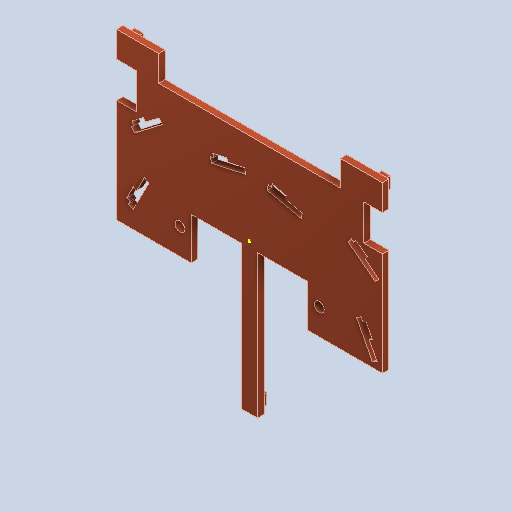
# Autodesk Inventor part: PCB
Saved by Autodesk Inventor 2022 (Build 260153000, 153)
## iProperties
Created: 2022-12-26
Part Number: PCB
Material: Copper
Document SubType Name: Modeling
Designer: Kamil
Density: 8.94 g/cm^3
Appearance: Copper - Satin
Author: Kamil
Autodesk Inventor part; units mm, degrees
(part 1 of 2)
ref_plane "YZ Plane" through (0, 0, 0) normal (1, 0, 0) x (0, 1, 0)
ref_plane "XZ Plane" through (0, 0, 0) normal (0, 1, 0) x (-1, 0, 0)
ref_plane "XY Plane" through (0, 0, 0) normal (0, 0, 1) x (1, 0, 0)
sketch "Sketch1" plane through (0, 0, 0) normal (0, 0, 1) x (1, 0, 0)
  circle A0 centre (-7.5, -8.85) radius 1.5 projected
  circle A1 centre (7.5, -8.85) radius 1.5 projected
  line L0 (50, 38.7074) -> (-50, 38.7074) projected
  line L1 (-50, 38.7074) -> (-50, -17.75) projected
  line L2 (-50, -17.75) -> (-15, -17.75) projected
  line L3 (-15, -17.75) -> (-15, -35.85) projected
  line L4 (-15, -35.85) -> (15, -35.85) projected
  line L5 (15, -35.85) -> (15, -17.75) projected
  line L6 (15, -17.75) -> (50, -17.75) projected
  line L7 (50, -17.75) -> (50, 38.7074) projected
  circle A2 centre (7.5, -26.85) radius 1.75 projected
  circle A3 centre (-7.5, -26.85) radius 1.75 projected
  line L8 (50, 31.0794) -> (-50, 31.0794) projected
  line L9 (25, 26.7074) -> (-25, 26.7074) projected
  line L10 (25, 31.0794) -> (25, 26.7074) projected
  line L11 (-25, 38.7074) -> (-25, 26.7074) projected
  line L12 (25, 26.7074) -> (25, 38.7074) projected
  line L13 (-15, -4.85) -> (-15, -48.05) projected
  line L14 (15, -4.85) -> (-15, -4.85) projected
  line L15 (15, -48.05) -> (15, -4.85) projected
  line L16 (44, 38.7074) -> (44, -17.75) projected
  line L17 (0, 26.7074) -> (0, -4.85)
  line L18 (-44, 38.7074) -> (-44, -17.75)
  point P0 (0, 0)
  constraints: 4 end point, 2 midpoint, 2 symmetric about line
extrude "Extrusion1" add sketch "Sketch1" along normal blind 2.4 contours L16 L8 L12 L0 | L16 L6 L15 L14 L17 L9 L10 L8 | L11 L8 L18 L0 | L11 L9 L17 L14 L13 L2 L18 L8
sketch "Sketch2" plane through (0, 0, 0) normal (0, 0, -1) x (-1, 0, 0)
  line L0 (-15, -4.85) -> (-15, -17.75) projected
  line L1 (-15, -17.75) -> (-44, -17.75) projected
  line L2 (-44, -17.75) -> (-44, 38.7074) projected
  line L3 (-44, 38.7074) -> (-25, 38.7074) projected
  line L4 (-25, 38.7074) -> (-25, 26.7074) projected
  line L5 (-25, 26.7074) -> (25, 26.7074) projected
  line L6 (25, 26.7074) -> (25, 38.7074) projected
  line L7 (25, 38.7074) -> (44, 38.7074) projected
  line L8 (44, 38.7074) -> (44, -17.75) projected
  line L9 (44, -17.75) -> (15, -17.75) projected
  line L10 (15, -17.75) -> (15, -4.85) projected
  line L11 (15, -4.85) -> (-15, -4.85) projected
  point P0 (0, 0)
extrude "Extrusion2" cut sketch "Sketch2" against normal blind 0.4
sketch "Sketch3" plane through (-44, -17.75, 2.4) normal (-1, 0, 0) x (0, 0, 1)
  line L0 (-2.4, 56.4574) -> (-5.4, 59.4574) projected
  line L1 (-5.4, 59.4574) -> (-5.4, 0) projected
  line L2 (-2.4, 0) -> (-5.4, 0) projected
  line L3 (-2.4, 56.4574) -> (-2.4, 0) projected
  line L4 (5.2279, 48.8294) -> (-7.5, 61.5574) projected
  line L5 (-2, 56.4574) -> (-2, 0) projected
  line L6 (-2, 0) -> (0, 0) projected
  line L7 (0, 56.4574) -> (0, 0) projected
  line L8 (-2, 56.4574) -> (0, 56.4574) projected
  line L9 (5.2279, 48.8294) -> (-2.4, 56.4574) projected
  line L10 (-2.4, 56.4574) -> (-2.4, 44.4574) projected
  line L11 (-2.4, 44.4574) -> (5.2279, 44.4574) projected
  line L12 (5.2279, 44.4574) -> (5.2279, 48.8294) projected
  line L13 (-2, 56.4574) -> (-2, 44.4574) projected
  line L14 (-2, 48.8294) -> (0, 48.8294)
  line L15 (0, 0) -> (0, 56.4574) projected
  line L16 (0, 50.4574) -> (-2, 50.4574)
  point P0 (-2.4, 17.75)
  constraints: 4 end point, 3 point on line, 1 midpoint, 1 perpendicular
extrude "Extrusion3" cut sketch "Sketch3" against normal through all contours L5 L8 L7 L4 | L4 L7 L16 L5
sketch "Sketch4" plane through (0, 0, 0.4) normal (0, 0, -1) x (-1, 0, 0)
  line L0 (-3.5, -4.85) -> (-3.5, -48.05) projected
  line L1 (3.5, -48.05) -> (3.5, -4.85) projected
  line L2 (5.6525, -48.05) -> (-5.6525, -48.05) projected
  line L3 (-44, 32.7074) -> (-25, 32.7074) projected
  line L4 (-25, 32.7074) -> (-25, 26.7074) projected
  line L5 (-25, 26.7074) -> (25, 26.7074) projected
  line L6 (25, 26.7074) -> (25, 32.7074) projected
  line L7 (25, 32.7074) -> (44, 32.7074) projected
  line L8 (44, 32.7074) -> (44, -17.75) projected
  line L9 (44, -17.75) -> (15, -17.75) projected
  line L10 (15, -17.75) -> (15, -4.85) projected
  line L11 (15, -4.85) -> (-15, -4.85) projected
  line L12 (-15, -4.85) -> (-15, -17.75) projected
  line L13 (-15, -17.75) -> (-44, -17.75) projected
  line L14 (-44, -17.75) -> (-44, 32.7074) projected
  point P0 (0, 0)
extrude "Extrusion4" add sketch "Sketch4" against normal blind 2 contours L11 L1 L2 L0
sketch "Sketch5" plane through (0, 0, 2.4) normal (0, 0, 1) x (1, 0, 0)
  line L0 (44, 32.7074) -> (25, 32.7074) projected
  line L1 (25, 32.7074) -> (25, 26.7074) projected
  line L2 (25, 26.7074) -> (-25, 26.7074) projected
  line L3 (-25, 26.7074) -> (-25, 32.7074) projected
  line L4 (-25, 32.7074) -> (-44, 32.7074) projected
  line L5 (-44, 32.7074) -> (-44, -17.75) projected
  line L6 (-44, -17.75) -> (-15, -17.75) projected
  line L7 (-15, -17.75) -> (-15, -4.85) projected
  line L8 (-15, -4.85) -> (-3.5, -4.85) projected
  line L9 (-3.5, -4.85) -> (-3.5, -48.05) projected
  line L10 (-3.5, -48.05) -> (3.5, -48.05) projected
  line L11 (3.5, -48.05) -> (3.5, -4.85) projected
  line L12 (3.5, -4.85) -> (15, -4.85) projected
  line L13 (15, -4.85) -> (15, -17.75) projected
  line L14 (15, -17.75) -> (44, -17.75) projected
  line L15 (44, -17.75) -> (44, 32.7074) projected
  line L16 (-25, 31.0794) -> (25, 31.0794) projected
  point P0 (0, 0)
extrude "Extrusion5" add sketch "Sketch5" against normal blind 2 contours L1 L2 L3 L16
sketch "Sketch6" plane through (0, 0, 2.4) normal (0, 0, 1) x (1, 0, 0)
  line L0 (44, 32.7074) -> (25, 32.7074) projected
  line L1 (25, 32.7074) -> (25, 31.0794) projected
  line L2 (25, 31.0794) -> (-25, 31.0794) projected
  line L3 (-25, 31.0794) -> (-25, 32.7074) projected
  line L4 (-25, 32.7074) -> (-44, 32.7074) projected
  line L5 (-44, 32.7074) -> (-44, -17.75) projected
  line L6 (-44, -17.75) -> (-15, -17.75) projected
  line L7 (-15, -17.75) -> (-15, -4.85) projected
  line L8 (-15, -4.85) -> (-3.5, -4.85) projected
  line L9 (-3.5, -4.85) -> (-3.5, -48.05) projected
  line L10 (-3.5, -48.05) -> (3.5, -48.05) projected
  line L11 (3.5, -48.05) -> (3.5, -4.85) projected
  line L12 (3.5, -4.85) -> (15, -4.85) projected
  line L13 (15, -4.85) -> (15, -17.75) projected
  line L14 (15, -17.75) -> (44, -17.75) projected
  line L15 (44, -17.75) -> (44, 32.7074) projected
  line L16 (25, 32.7074) -> (25, 31.0794) projected
  line L17 (25, 32.7074) -> (44, 32.7074)
  line L18 (44, 32.7074) -> (44, 36.1074)
  line L19 (44, 36.1074) -> (25, 36.1074)
  line L20 (25, 36.1074) -> (25, 32.7074)
  line L21 (-44, 32.7074) -> (-25, 32.7074) projected
  line L22 (-44, 32.7074) -> (-25, 32.7074)
  line L23 (-25, 32.7074) -> (-25, 36.1074)
  line L24 (-25, 36.1074) -> (-44, 36.1074)
  line L25 (-44, 36.1074) -> (-44, 32.7074)
  point P0 (0, 0)
  dimension "d10" = 3.4
  constraints: 16 end point, 4 parallel, 2 horizontal, 2 perpendicular, 1 point on line
  measures "d10" distance of L18.end L17.end
extrude "Extrusion6" add sketch "Sketch6" against normal blind 2 contours L0 L20 L19 L18 | L4 L25 L24 L23
sketch "Sketch9" plane through (0, 0, 2.4) normal (0, 0, 1) x (1, 0, 0)
  line L0 (44, -17.75) -> (44, 36.1074) projected
  line L1 (44, 33.1074) -> (44, 36.1074)
  line L2 (15, -17.75) -> (44, -17.75) projected
  line L3 (44, 36.1074) -> (41, 36.1074)
  line L4 (41, 36.1074) -> (41, -17.75)
  line L5 (41, -17.75) -> (44, -17.75)
  line L6 (44, -17.75) -> (44, 36.1074)
  line L7 (-44, 36.1074) -> (-44, -17.75) projected
  line L8 (44, -17.75) -> (-44, -17.75)
  line L9 (-44, -17.75) -> (-44, -13.0168)
  line L10 (-44, -13.0168) -> (44, -13.0168)
  line L11 (44, -13.0168) -> (44, -17.75)
  line L12 (15, -4.85) -> (15, -17.75) projected
  line L13 (15, -17.75) -> (18, -17.75)
  line L14 (18, -17.75) -> (18, -4.85)
  line L15 (18, -4.85) -> (15, -4.85)
  line L16 (15, -4.85) -> (15, -17.75)
  line L17 (-15, -17.75) -> (-15, -4.85) projected
  line L18 (-15, -17.75) -> (-18, -17.75)
  line L19 (-18, -17.75) -> (-18, -4.85)
  line L20 (-18, -4.85) -> (-15, -4.85)
  line L21 (-15, -4.85) -> (-15, -17.75)
  line L22 (-25, 36.1074) -> (-44, 36.1074) projected
  line L23 (-44, -17.75) -> (-41, -17.75)
  line L24 (-41, -17.75) -> (-41, 36.1074)
  line L25 (-41, 36.1074) -> (-44, 36.1074)
  line L26 (-44, 36.1074) -> (-44, -17.75)
  line L27 (25, 36.1074) -> (25, 31.0794) projected
  line L28 (25, 36.1074) -> (28, 36.1074)
  line L29 (28, 36.1074) -> (28, 31.0794)
  line L30 (28, 31.0794) -> (25, 31.0794)
  line L31 (25, 31.0794) -> (25, 36.1074)
  line L32 (-25, 36.1074) -> (-28, 36.1074)
  line L33 (-28, 36.1074) -> (-28, 31.0794)
  line L34 (-28, 31.0794) -> (-25, 31.0794)
  line L35 (-25, 31.0794) -> (-25, 36.1074)
  line L36 (-18, -4.85) -> (-3.5, -4.85)
  line L37 (-3.5, -4.85) -> (-3.5, -1.85)
  line L38 (-3.5, -1.85) -> (-18, -1.85)
  line L39 (-18, -1.85) -> (-18, -4.85)
  line L40 (3.5, -48.05) -> (3.5, -4.85) projected
  line L41 (3.5, -4.85) -> (18, -4.85)
  line L42 (18, -4.85) -> (18, -1.85)
  line L43 (18, -1.85) -> (3.5, -1.85)
  line L44 (3.5, -1.85) -> (3.5, -4.85)
  line L45 (-3.5, -48.05) -> (3.5, -48.05) projected
  line L46 (3.5, -1.85) -> (2.5, -1.85)
  line L47 (2.5, -1.85) -> (2.5, -48.05)
  line L48 (2.5, -48.05) -> (3.5, -48.05)
  line L49 (3.5, -48.05) -> (3.5, -1.85)
  line L50 (-3.5, -48.05) -> (-2.5, -48.05)
  line L51 (-2.5, -48.05) -> (-2.5, -4.85)
  line L52 (-2.5, -4.85) -> (-3.5, -4.85)
  line L53 (-3.5, -4.85) -> (-3.5, -48.05)
  line L54 (-28, 31.0794) -> (28, 31.0794)
  line L55 (28, 31.0794) -> (28, 28.0794)
  line L56 (28, 28.0794) -> (-28, 28.0794)
  line L57 (-28, 28.0794) -> (-28, 31.0794)
  point P0 (0, 0)
  point P1 (-18, -13.0168)
  point P2 (-41, -13.0168)
  point P3 (41, -13.0168)
  point P4 (18, -13.0168)
  dimension "d14" = 3
  dimension "d15" = 3
  dimension "d16" = 3
  dimension "d17" = 3
  dimension "d18" = 3
  dimension "d19" = 3
  dimension "d20" = 3
  dimension "d21" = 1
  dimension "d22" = 1
  dimension "d23" = 3
  constraints: 98 end point, 24 parallel, 12 horizontal, 12 perpendicular, 9 point on line
  measures "d14" distance of L5.end L4.end
  measures "d15" distance of L15.end L14.end
  measures "d16" distance of L19.end L20.end
  measures "d17" distance of L25.end L24.end
  measures "d18" distance of L29.end L30.end
  measures "d19" distance of L34.end L33.end
  measures "d20" distance of L37.end L36.end
  measures "d21" distance of L48.end L47.end
  measures "d22" distance of L52.end L51.end
  measures "d23" distance of L54.end L55.end
extrude "Extrusion7" cut sketch "Sketch9" against normal blind 2 contours L2 L4 L10 L0 | L22 L35 L34 L33 | L10 L4 L3 L0 | L2 L14 L10 L4 | L2 L12 L10 L14 | L10 L12 L15 L14 | L15 L41 L44 L43 L42 | L40 L45 L47 L8 | L8 L47 L10 L40 | L10 L47 L46 L44 L40 | L51 L45 L53 L8 | L8 L53 L10 L51 | L10 L53 L52 L51 | L8 L19 L10 L17 | L10 L19 L20 L17 | L36 L20 L39 L38 L37 | L8 L24 L10 L19 | L8 L7 L10 L24 | L10 L7 L22 L24 | L34 L54 L30 L55 L56 L57 | L27 L28 L29 L30
sketch "Sketch8" plane through (0, 0, 2.4) normal (0, 0, 1) x (1, 0, 0)
  line L0 (-40.8006, -12.2713) -> (-38.4785, -1.8263)
  line L1 (-40.8006, -12.2713) -> (-39.2388, -12.6185)
  line L2 (-36.9167, -2.1735) -> (-39.2388, -12.6185)
  line L3 (-38.4785, -1.8263) -> (-36.9167, -2.1735)
  line L4 (36.1788, 2.3275) -> (38.4885, -8.1203)
  line L5 (36.1788, 2.3275) -> (34.6166, 1.9821)
  line L6 (36.9263, -8.4656) -> (34.6166, 1.9821)
  line L7 (38.4885, -8.1203) -> (36.9263, -8.4656)
  line L8 (-3.9031, 21.0008) -> (-14.3503, 18.6891)
  line L9 (-3.9031, 21.0008) -> (-3.5574, 19.4386)
  line L10 (-14.0047, 17.1269) -> (-3.5574, 19.4386)
  line L11 (-14.3503, 18.6891) -> (-14.0047, 17.1269)
  line L12 (9.235, 18.6922) -> (-1.2105, 21.0122)
  line L13 (9.235, 18.6922) -> (8.888, 17.1302)
  line L14 (-1.5574, 19.4503) -> (8.888, 17.1302)
  line L15 (-1.2105, 21.0122) -> (-1.5574, 19.4503)
  line L16 (-39.7739, 3.0399) -> (-32.2458, 10.6437)
  line L17 (-39.7739, 3.0399) -> (-38.6369, 1.9142)
  line L18 (-31.1088, 9.5181) -> (-38.6369, 1.9142)
  line L19 (-32.2458, 10.6437) -> (-31.1088, 9.5181)
  line L20 (32.5559, 15.107) -> (40.1958, 7.6154)
  line L21 (32.5559, 15.107) -> (31.4357, 13.9645)
  line L22 (39.0755, 6.473) -> (31.4357, 13.9645)
  line L23 (40.1958, 7.6154) -> (39.0755, 6.473)
  line L24 (25, 36.1074) -> (25, 31.0794)
  line L25 (25, 31.0794) -> (-25, 31.0794)
  line L26 (-25, 31.0794) -> (-25, 36.1074)
  line L27 (-25, 36.1074) -> (-44, 36.1074)
  line L28 (-44, 36.1074) -> (-44, -17.75)
  line L29 (-44, -17.75) -> (-15, -17.75)
  line L30 (-15, -17.75) -> (-15, -4.85)
  line L31 (-15, -4.85) -> (-3.5, -4.85)
  line L32 (-3.5, -4.85) -> (-3.5, -48.05)
  line L33 (-3.5, -48.05) -> (3.5, -48.05)
  line L34 (3.5, -48.05) -> (3.5, -4.85)
  line L35 (3.5, -4.85) -> (15, -4.85)
  line L36 (15, -4.85) -> (15, -17.75)
  line L37 (15, -17.75) -> (44, -17.75)
  line L38 (44, -17.75) -> (44, 36.1074)
  line L39 (44, 36.1074) -> (25, 36.1074)
  point P0 (0, 0)
extrude "Extrusion8" add sketch "Sketch8" along normal blind 14 contours L0 L3 L2 L1 | L4 L7 L6 L5 | L9 L10 L11 L8 | L13 L14 L15 L12 | L16 L19 L18 L17 | L20 L23 L22 L21
sketch "Sketch10" plane through (0, 0, 2.4) normal (0, 0, 1) x (1, 0, 0)
  line L0 (-1.2105, 21.0122) -> (9.235, 18.6922) projected
  line L1 (9.235, 18.6922) -> (8.888, 17.1302) projected
  line L2 (8.888, 17.1302) -> (-1.5574, 19.4503) projected
  line L3 (-1.5574, 19.4503) -> (-1.2105, 21.0122) projected
  line L4 (-39.2388, -12.6185) -> (-40.8006, -12.2713) projected
  line L5 (-40.8006, -12.2713) -> (-38.4785, -1.8263) projected
  line L6 (-38.4785, -1.8263) -> (-36.9167, -2.1735) projected
  line L7 (-36.9167, -2.1735) -> (-39.2388, -12.6185) projected
  line L8 (34.6166, 1.9821) -> (36.1788, 2.3275) projected
  line L9 (36.1788, 2.3275) -> (38.4885, -8.1203) projected
  line L10 (38.4885, -8.1203) -> (36.9263, -8.4656) projected
  line L11 (36.9263, -8.4656) -> (34.6166, 1.9821) projected
  line L12 (-14.3503, 18.6891) -> (-3.9031, 21.0008) projected
  line L13 (-3.9031, 21.0008) -> (-3.5574, 19.4386) projected
  line L14 (-3.5574, 19.4386) -> (-14.0047, 17.1269) projected
  line L15 (-14.0047, 17.1269) -> (-14.3503, 18.6891) projected
  line L16 (-38.6369, 1.9142) -> (-39.7739, 3.0399) projected
  line L17 (-39.7739, 3.0399) -> (-32.2458, 10.6437) projected
  line L18 (-32.2458, 10.6437) -> (-31.1088, 9.5181) projected
  line L19 (-31.1088, 9.5181) -> (-38.6369, 1.9142) projected
  line L20 (31.4357, 13.9645) -> (32.5559, 15.107) projected
  line L21 (32.5559, 15.107) -> (40.1958, 7.6154) projected
  line L22 (40.1958, 7.6154) -> (39.0755, 6.473) projected
  line L23 (39.0755, 6.473) -> (31.4357, 13.9645) projected
  line L24 (28, 36.1074) -> (28, 28.0794) projected
  line L25 (28, 28.0794) -> (-28, 28.0794) projected
  line L26 (-28, 28.0794) -> (-28, 36.1074) projected
  line L27 (-28, 36.1074) -> (-41, 36.1074) projected
  line L28 (-41, 36.1074) -> (-41, -13.0168) projected
  line L29 (-41, -13.0168) -> (-18, -13.0168) projected
  line L30 (-18, -13.0168) -> (-18, -1.85) projected
  line L31 (-18, -1.85) -> (-3.5, -1.85) projected
  line L32 (-3.5, -1.85) -> (-3.5, -4.85) projected
  line L33 (-3.5, -4.85) -> (-2.5, -4.85) projected
  line L34 (-2.5, -4.85) -> (-2.5, -48.05) projected
  line L35 (-2.5, -48.05) -> (2.5, -48.05) projected
  line L36 (2.5, -48.05) -> (2.5, -1.85) projected
  line L37 (2.5, -1.85) -> (18, -1.85) projected
  line L38 (18, -1.85) -> (18, -13.0168) projected
  line L39 (18, -13.0168) -> (41, -13.0168) projected
  line L40 (41, -13.0168) -> (41, 36.1074) projected
  line L41 (41, 36.1074) -> (28, 36.1074) projected
  line L42 (-3.5, -4.85) -> (-2.5, -4.85)
  line L43 (-2.5, -4.85) -> (-2.5, -1.85)
  line L44 (-2.5, -1.85) -> (-3.5, -1.85)
  line L45 (-3.5, -1.85) -> (-3.5, -4.85)
  point P0 (0, 0)
  constraints: 8 end point, 2 parallel, 1 horizontal, 1 perpendicular
extrude "Extrusion9" cut sketch "Sketch10" against normal blind 14 contours L44 L43 L33 L32
sketch "Sketch11" plane through (0, 0, 2.4) normal (0, 0, 1) x (1, 0, 0)
  line L0 (-2.5, -1.85) -> (-2.5, -48.05) projected
  line L1 (-2.5, -48.05) -> (2.5, -48.05) projected
  line L2 (2.5, -48.05) -> (2.5, -1.85) projected
  line L3 (2.5, -1.85) -> (18, -1.85) projected
  line L4 (18, -1.85) -> (18, -13.0168) projected
  line L5 (18, -13.0168) -> (41, -13.0168) projected
  line L6 (41, -13.0168) -> (41, 36.1074) projected
  line L7 (41, 36.1074) -> (28, 36.1074) projected
  line L8 (28, 36.1074) -> (28, 28.0794) projected
  line L9 (28, 28.0794) -> (-28, 28.0794) projected
  line L10 (-28, 28.0794) -> (-28, 36.1074) projected
  line L11 (-28, 36.1074) -> (-41, 36.1074) projected
  line L12 (-41, 36.1074) -> (-41, -13.0168) projected
  line L13 (-41, -13.0168) -> (-18, -13.0168) projected
  line L14 (-18, -13.0168) -> (-18, -1.85) projected
  line L15 (-18, -1.85) -> (-2.5, -1.85) projected
  line L16 (-1.2105, 21.0122) -> (9.235, 18.6922) projected
  line L17 (9.235, 18.6922) -> (8.888, 17.1302) projected
  line L18 (8.888, 17.1302) -> (-1.5574, 19.4503) projected
  line L19 (-1.5574, 19.4503) -> (-1.2105, 21.0122) projected
  line L20 (-39.2388, -12.6185) -> (-40.8006, -12.2713) projected
  line L21 (-40.8006, -12.2713) -> (-38.4785, -1.8263) projected
  line L22 (-38.4785, -1.8263) -> (-36.9167, -2.1735) projected
  line L23 (-36.9167, -2.1735) -> (-39.2388, -12.6185) projected
  line L24 (34.6166, 1.9821) -> (36.1788, 2.3275) projected
  line L25 (36.1788, 2.3275) -> (38.4885, -8.1203) projected
  line L26 (38.4885, -8.1203) -> (36.9263, -8.4656) projected
  line L27 (36.9263, -8.4656) -> (34.6166, 1.9821) projected
  line L28 (-14.3503, 18.6891) -> (-3.9031, 21.0008) projected
  line L29 (-3.9031, 21.0008) -> (-3.5574, 19.4386) projected
  line L30 (-3.5574, 19.4386) -> (-14.0047, 17.1269) projected
  line L31 (-14.0047, 17.1269) -> (-14.3503, 18.6891) projected
  line L32 (-38.6369, 1.9142) -> (-39.7739, 3.0399) projected
  line L33 (-39.7739, 3.0399) -> (-32.2458, 10.6437) projected
  line L34 (-32.2458, 10.6437) -> (-31.1088, 9.5181) projected
  line L35 (-31.1088, 9.5181) -> (-38.6369, 1.9142) projected
  line L36 (31.4357, 13.9645) -> (32.5559, 15.107) projected
  line L37 (32.5559, 15.107) -> (40.1958, 7.6154) projected
  line L38 (40.1958, 7.6154) -> (39.0755, 6.473) projected
  line L39 (39.0755, 6.473) -> (31.4357, 13.9645) projected
  line L40 (0, -48.05) -> (0, 28.0794)
  line L41 (28, 28.0794) -> (-28, 28.0794) projected
  line L42 (41, -13.0168) -> (41, 36.1074) projected
  line L43 (41, 28.0794) -> (35.2556, 28.0794)
  line L44 (35.2556, 28.0794) -> (35.2556, 17.8601)
  line L45 (35.2556, 17.8601) -> (41, 17.8601)
  line L46 (41, 17.8601) -> (41, 28.0794)
  line L47 (-41, 28.0794) -> (-35.2556, 28.0794)
  line L48 (-35.2556, 28.0794) -> (-35.2556, 17.8601)
  line L49 (-35.2556, 17.8601) -> (-41, 17.8601)
  point P0 (0, 0)
  constraints: 16 end point, 4 symmetric about line, 2 midpoint, 2 parallel, 1 horizontal, 1 perpendicular, 1 point on line
extrude "Extrusion10" cut sketch "Sketch11" against normal blind 14 contours L12 L47 L48 L49 | L45 L44 L43 L6
sketch "Sketch12" plane through (0, 0, 2.4) normal (0, 0, 1) x (1, 0, 0)
  line L0 (31.4357, 13.9645) -> (32.5559, 15.107) projected
  line L1 (32.5559, 15.107) -> (40.1958, 7.6154) projected
  line L2 (40.1958, 7.6154) -> (39.0755, 6.473) projected
  line L3 (39.0755, 6.473) -> (31.4357, 13.9645) projected
  line L4 (-38.6369, 1.9142) -> (-39.7739, 3.0399) projected
  line L5 (-39.7739, 3.0399) -> (-32.2458, 10.6437) projected
  line L6 (-32.2458, 10.6437) -> (-31.1088, 9.5181) projected
  line L7 (-31.1088, 9.5181) -> (-38.6369, 1.9142) projected
  line L8 (-14.3503, 18.6891) -> (-3.9031, 21.0008) projected
  line L9 (-3.9031, 21.0008) -> (-3.5574, 19.4386) projected
  line L10 (-3.5574, 19.4386) -> (-14.0047, 17.1269) projected
  line L11 (-14.0047, 17.1269) -> (-14.3503, 18.6891) projected
  line L12 (34.6166, 1.9821) -> (36.1788, 2.3275) projected
  line L13 (36.1788, 2.3275) -> (38.4885, -8.1203) projected
  line L14 (38.4885, -8.1203) -> (36.9263, -8.4656) projected
  line L15 (36.9263, -8.4656) -> (34.6166, 1.9821) projected
  line L16 (-39.2388, -12.6185) -> (-40.8006, -12.2713) projected
  line L17 (-40.8006, -12.2713) -> (-38.4785, -1.8263) projected
  line L18 (-38.4785, -1.8263) -> (-36.9167, -2.1735) projected
  line L19 (-36.9167, -2.1735) -> (-39.2388, -12.6185) projected
  line L20 (-1.2105, 21.0122) -> (9.235, 18.6922) projected
  line L21 (9.235, 18.6922) -> (8.888, 17.1302) projected
  line L22 (8.888, 17.1302) -> (-1.5574, 19.4503) projected
  line L23 (-1.5574, 19.4503) -> (-1.2105, 21.0122) projected
  line L24 (-41, 28.0794) -> (-35.2556, 28.0794) projected
  line L25 (-35.2556, 28.0794) -> (-35.2556, 17.8601) projected
  line L26 (-35.2556, 17.8601) -> (-41, 17.8601) projected
  line L27 (-41, 17.8601) -> (-41, -13.0168) projected
  line L28 (-41, -13.0168) -> (-18, -13.0168) projected
  line L29 (-18, -13.0168) -> (-18, -1.85) projected
  line L30 (-18, -1.85) -> (-2.5, -1.85) projected
  line L31 (-2.5, -1.85) -> (-2.5, -48.05) projected
  line L32 (-2.5, -48.05) -> (2.5, -48.05) projected
  line L33 (2.5, -48.05) -> (2.5, -1.85) projected
  line L34 (2.5, -1.85) -> (18, -1.85) projected
  line L35 (18, -1.85) -> (18, -13.0168) projected
  line L36 (18, -13.0168) -> (41, -13.0168) projected
  line L37 (41, -13.0168) -> (41, 17.8601) projected
  line L38 (41, 17.8601) -> (35.2556, 17.8601) projected
  line L39 (35.2556, 17.8601) -> (35.2556, 28.0794) projected
  line L40 (35.2556, 28.0794) -> (41, 28.0794) projected
  line L41 (41, 28.0794) -> (41, 36.1074) projected
  line L42 (41, 36.1074) -> (28, 36.1074) projected
  line L43 (28, 36.1074) -> (28, 28.0794) projected
  line L44 (28, 28.0794) -> (-28, 28.0794) projected
  line L45 (-28, 28.0794) -> (-28, 36.1074) projected
  line L46 (-28, 36.1074) -> (-41, 36.1074) projected
  line L47 (-41, 36.1074) -> (-41, 28.0794) projected
  line L48 (-1.5574, 19.4503) -> (-1.2105, 21.0122) projected
  line L49 (-1.5574, 19.4503) -> (-1.5574, 15.4503)
  line L50 (-1.5574, 19.4503) -> (8.888, 17.1302) projected
  line L51 (9.235, 18.6922) -> (-1.2105, 21.0122) projected
  line L52 (-1.2105, 21.0122) -> (-1.5574, 19.4503) projected
  line L53 (-1.5574, 19.4503) -> (8.888, 17.1302) projected
  line L54 (8.888, 17.1302) -> (9.235, 18.6922) projected
  line L55 (9.235, 18.6922) -> (-1.2105, 21.0122) projected
  line L56 (-14.3503, 18.6891) -> (-14.0047, 17.1269) projected
  line L57 (-14.0047, 17.1269) -> (-3.5574, 19.4386) projected
  line L58 (-3.5574, 19.4386) -> (-3.9031, 21.0008) projected
  line L59 (-3.9031, 21.0008) -> (-14.3503, 18.6891) projected
  line L60 (-1.5574, 17.4503) -> (8.888, 15.1302)
  line L61 (9.235, 18.6922) -> (8.888, 17.1302) projected
  line L62 (-1.2105, 21.0122) -> (9.235, 18.6922) projected
  line L63 (9.235, 16.6922) -> (-1.2105, 19.0122)
  line L64 (-1.2105, 19.0122) -> (-1.5574, 17.4503)
  line L65 (-3.9031, 21.0008) -> (-3.5574, 19.4386) projected
  line L66 (-14.0047, 17.1269) -> (-14.3503, 18.6891) projected
  line L67 (-3.9031, 19.0008) -> (-14.3503, 16.6891)
  line L68 (-14.3503, 16.6891) -> (-14.0047, 15.1269)
  line L69 (-14.0047, 15.1269) -> (-3.5574, 17.4386)
  line L70 (-3.5574, 19.4386) -> (-14.0047, 17.1269) projected
  line L71 (-3.5574, 17.4386) -> (-3.9031, 19.0008)
  line L72 (8.888, 15.1302) -> (9.235, 16.6922)
  line L73 (12.4945, 18.6922) -> (12.4945, 16.6922)
  point P0 (0, 0)
  point P1 (-3.5574, 17.4386)
  dimension "d33" = 2
  constraints: 20 end point, 4 perpendicular, 3 parallel, 2 vertical
  measures "d33" distance of L73.start L73.end
extrude "Extrusion11" add sketch "Sketch12" along normal blind 14 contours L64 L63 L72 L60 | L71 L69 L68 L67
extrude "Extrusion12" cut sketch "Sketch12" along normal blind 14 contours L8 L9 L10 L11 | L20 L21 L22 L23
sketch "Sketch13" plane through (0, 0, 0.4) normal (0, 0, -1) x (-1, 0, 0)
  line L0 (41, 17.8601) -> (35.2556, 17.8601) projected
  line L1 (35.2556, 17.8601) -> (35.2556, 28.0794) projected
  line L2 (35.2556, 28.0794) -> (41, 28.0794) projected
  line L3 (41, 28.0794) -> (41, 36.1074) projected
  line L4 (41, 36.1074) -> (28, 36.1074) projected
  line L5 (28, 36.1074) -> (28, 28.0794) projected
  line L6 (28, 28.0794) -> (-28, 28.0794) projected
  line L7 (-28, 28.0794) -> (-28, 36.1074) projected
  line L8 (-28, 36.1074) -> (-41, 36.1074) projected
  line L9 (-41, 36.1074) -> (-41, 28.0794) projected
  line L10 (-41, 28.0794) -> (-35.2556, 28.0794) projected
  line L11 (-35.2556, 28.0794) -> (-35.2556, 17.8601) projected
  line L12 (-35.2556, 17.8601) -> (-41, 17.8601) projected
  line L13 (-41, 17.8601) -> (-41, -13.0168) projected
  line L14 (-41, -13.0168) -> (-18, -13.0168) projected
  line L15 (-18, -13.0168) -> (-18, -1.85) projected
  line L16 (-18, -1.85) -> (-2.5, -1.85) projected
  line L17 (-2.5, -1.85) -> (-2.5, -48.05) projected
  line L18 (-2.5, -48.05) -> (2.5, -48.05) projected
  line L19 (2.5, -48.05) -> (2.5, -1.85) projected
  line L20 (2.5, -1.85) -> (18, -1.85) projected
  line L21 (18, -1.85) -> (18, -13.0168) projected
  line L22 (18, -13.0168) -> (41, -13.0168) projected
  line L23 (41, -13.0168) -> (41, 17.8601) projected
  line L24 (2.5, -1.85) -> (2.5, -48.05) projected
  line L25 (-2.5, -48.05) -> (2.5, -48.05)
  line L26 (2.5, -48.05) -> (2.5, -46.05)
  line L27 (2.5, -46.05) -> (-2.5, -46.05)
  line L28 (-2.5, -46.05) -> (-2.5, -48.05)
  point P0 (0, 0)
  dimension "d38" = 2
  constraints: 8 end point, 2 parallel, 1 horizontal, 1 perpendicular, 1 point on line
  measures "d38" distance of L26.end L25.end
extrude "Extrusion13" cut sketch "Sketch13" against normal blind 14 contours L19 L18 L17 L27
sketch "Sketch14" plane through (0, 0, 2.4) normal (0, 0, 1) x (1, 0, 0)
  circle A0 centre (21.5, -6.85) radius 1.5 projected
  circle A1 centre (-21.5, -6.85) radius 1.5 projected
  circle A2 centre (7.5, -24.85) radius 1.75 projected
  circle A3 centre (-7.5, -24.85) radius 1.75 projected
  circle A4 centre (7.5, -6.85) radius 1.5 projected
  circle A5 centre (-7.5, -6.85) radius 1.5 projected
  line L0 (-50, 42.8801) -> (50, 42.8801) projected
  line L1 (50, -15.75) -> (50, 42.8801) projected
  line L2 (15, -15.75) -> (50, -15.75) projected
  line L3 (15, -33.85) -> (15, -15.75) projected
  line L4 (15, -33.85) -> (-15, -33.85) projected
  line L5 (-15, -15.75) -> (-15, -33.85) projected
  line L6 (-50, -15.75) -> (-15, -15.75) projected
  line L7 (-50, 42.8801) -> (-50, -15.75) projected
  point P0 (0, 0)
extrude "Extrusion14" cut sketch "Sketch14" against normal blind 14 contours A0 | A1
sketch "Sketch15" plane through (0, 0, 0.4) normal (0, 0, -1) x (-1, 0, 0)
  circle A0 centre (21.5, -6.85) radius 1.5 projected
  circle A1 centre (-21.5, -6.85) radius 1.5 projected
  line L0 (-2.5, -46.05) -> (2.5, -46.05) projected
  line L1 (2.5, -46.05) -> (2.5, -1.85) projected
  line L2 (2.5, -1.85) -> (18, -1.85) projected
  line L3 (18, -1.85) -> (18, -13.0168) projected
  line L4 (18, -13.0168) -> (41, -13.0168) projected
  line L5 (41, -13.0168) -> (41, 17.8601) projected
  line L6 (41, 17.8601) -> (35.2556, 17.8601) projected
  line L7 (35.2556, 17.8601) -> (35.2556, 28.0794) projected
  line L8 (35.2556, 28.0794) -> (41, 28.0794) projected
  line L9 (41, 28.0794) -> (41, 36.1074) projected
  line L10 (41, 36.1074) -> (28, 36.1074) projected
  line L11 (28, 36.1074) -> (28, 28.0794) projected
  line L12 (28, 28.0794) -> (-28, 28.0794) projected
  line L13 (-28, 28.0794) -> (-28, 36.1074) projected
  line L14 (-28, 36.1074) -> (-41, 36.1074) projected
  line L15 (-41, 36.1074) -> (-41, 28.0794) projected
  line L16 (-41, 28.0794) -> (-35.2556, 28.0794) projected
  line L17 (-35.2556, 28.0794) -> (-35.2556, 17.8601) projected
  line L18 (-35.2556, 17.8601) -> (-41, 17.8601) projected
  line L19 (-41, 17.8601) -> (-41, -13.0168) projected
  line L20 (-41, -13.0168) -> (-18, -13.0168) projected
  line L21 (-18, -13.0168) -> (-18, -1.85) projected
  line L22 (-18, -1.85) -> (-2.5, -1.85) projected
  line L23 (-2.5, -1.85) -> (-2.5, -46.05) projected
  line L24 (41, 28.0794) -> (41, 36.1074) projected
  line L25 (28, 36.1074) -> (28, 28.0794) projected
  line L26 (35.2556, 28.0794) -> (41, 28.0794) projected
  line L27 (39.4778, 35.1973) -> (36.7778, 35.1973)
  line L28 (36.7778, 35.1973) -> (36.7778, 31.7973)
  line L29 (36.7778, 31.7973) -> (39.4778, 31.7973)
  line L30 (39.4778, 31.7973) -> (39.4778, 35.1973)
  line L31 (1.35, -41.7382) -> (-1.35, -41.7382)
  line L32 (-1.35, -41.7382) -> (-1.35, -45.1382)
  line L33 (-1.35, -45.1382) -> (1.35, -45.1382)
  line L34 (1.35, -45.1382) -> (1.35, -41.7382)
  line L35 (-2.5, -46.05) -> (2.5, -46.05) projected
  line L36 (0, -46.05) -> (0, -32.5838)
  line L37 (38.1278, 28.0794) -> (38.1278, 36.1074)
  line L38 (41, 36.1074) -> (28, 36.1074) projected
  line L39 (-39.4778, 35.1973) -> (-36.7778, 35.1973)
  line L40 (-36.7778, 35.1973) -> (-36.7778, 31.7973)
  line L41 (-36.7778, 31.7973) -> (-39.4778, 31.7973)
  line L42 (-39.4778, 31.7973) -> (-39.4778, 35.1973)
  point P0 (0, 0)
  point P1 (38.1278, 32.0934)
  point P2 (38.1278, 32.0934)
  point P3 (0, -45.1382)
  point P4 (0, -45.1382)
  point P5 (38.1278, 34.5901)
  point P6 (38.1278, 35.1973)
  point P7 (38.1278, 35.1973)
  point P8 (-38.1278, 35.1973)
  dimension "d43" = 2.7
  dimension "d44" = 3.4
  dimension "d45" = 2.7
  dimension "d46" = 3.4
  constraints: 28 end point, 5 symmetric about line, 4 midpoint, 4 parallel, 4 point on line, 2 horizontal, 2 perpendicular, 2 vertical
  measures "d43" distance of L29.end L28.end
  measures "d44" distance of L28.end L27.end
  measures "d45" distance of L33.end L32.end
  measures "d46" distance of L32.end L32.start
extrude "Extrusion15" add sketch "Sketch15" along normal blind 2 contours L33 L32 L31 L36 | L36 L31 L34 L33 | L37 L27 L30 L29 | L29 L28 L27 L37 | L39 L40 L41 L42
sketch "Sketch16" plane through (0, 0, 16.4) normal (0, 0, 1) x (1, 0, 0)
  line L0 (31.4357, 13.9645) -> (39.0755, 6.473) projected
  line L1 (39.0755, 6.473) -> (40.1958, 7.6154) projected
  line L2 (40.1958, 7.6154) -> (32.5559, 15.107) projected
  line L3 (32.5559, 15.107) -> (31.4357, 13.9645) projected
  line L4 (34.6166, 1.9821) -> (36.9263, -8.4656) projected
  line L5 (36.9263, -8.4656) -> (38.4885, -8.1203) projected
  line L6 (38.4885, -8.1203) -> (36.1788, 2.3275) projected
  line L7 (36.1788, 2.3275) -> (34.6166, 1.9821) projected
  line L8 (-14.3503, 16.6891) -> (-14.0047, 15.1269) projected
  line L9 (-14.0047, 15.1269) -> (-3.5574, 17.4386) projected
  line L10 (-3.5574, 17.4386) -> (-3.9031, 19.0008) projected
  line L11 (-3.9031, 19.0008) -> (-14.3503, 16.6891) projected
  line L12 (-1.2105, 19.0122) -> (-1.5574, 17.4503) projected
  line L13 (-1.5574, 17.4503) -> (8.888, 15.1302) projected
  line L14 (8.888, 15.1302) -> (9.235, 16.6922) projected
  line L15 (9.235, 16.6922) -> (-1.2105, 19.0122) projected
  line L16 (-38.6369, 1.9142) -> (-31.1088, 9.5181) projected
  line L17 (-31.1088, 9.5181) -> (-32.2458, 10.6437) projected
  line L18 (-32.2458, 10.6437) -> (-39.7739, 3.0399) projected
  line L19 (-39.7739, 3.0399) -> (-38.6369, 1.9142) projected
  line L20 (-38.4785, -1.8263) -> (-40.8006, -12.2713) projected
  line L21 (-39.2388, -12.6185) -> (-36.9167, -2.1735) projected
  line L22 (-36.9167, -2.1735) -> (-38.4785, -1.8263) projected
  line L23 (-38.4785, -1.8263) -> (-40.8006, -12.2713) projected
  line L24 (-40.8006, -12.2713) -> (-39.2388, -12.6185) projected
  point P0 (0, 0)
extrude "Extrusion16" cut sketch "Sketch16" against normal through all
sketch "Sketch17" plane through (0, 0, 2.4) normal (0, 0, 1) x (1, 0, 0)
  circle A0 centre (-21.5, -6.85) radius 1.5 projected
  circle A1 centre (21.5, -6.85) radius 1.5 projected
  line L0 (-2.5, -46.05) -> (2.5, -46.05) projected
  line L1 (2.5, -46.05) -> (2.5, -1.85) projected
  line L2 (2.5, -1.85) -> (18, -1.85) projected
  line L3 (18, -1.85) -> (18, -13.0168) projected
  line L4 (18, -13.0168) -> (41, -13.0168) projected
  line L5 (41, -13.0168) -> (41, 17.8601) projected
  line L6 (41, 17.8601) -> (35.2556, 17.8601) projected
  line L7 (35.2556, 17.8601) -> (35.2556, 28.0794) projected
  line L8 (35.2556, 28.0794) -> (41, 28.0794) projected
  line L9 (41, 28.0794) -> (41, 36.1074) projected
  line L10 (41, 36.1074) -> (28, 36.1074) projected
  line L11 (28, 36.1074) -> (28, 28.0794) projected
  line L12 (28, 28.0794) -> (-28, 28.0794) projected
  line L13 (-28, 28.0794) -> (-28, 36.1074) projected
  line L14 (-28, 36.1074) -> (-41, 36.1074) projected
  line L15 (-41, 36.1074) -> (-41, 28.0794) projected
  line L16 (-41, 28.0794) -> (-35.2556, 28.0794) projected
  line L17 (-35.2556, 28.0794) -> (-35.2556, 17.8601) projected
  line L18 (-35.2556, 17.8601) -> (-41, 17.8601) projected
  line L19 (-41, 17.8601) -> (-41, -13.0168) projected
  line L20 (-41, -13.0168) -> (-18, -13.0168) projected
  line L21 (-18, -13.0168) -> (-18, -1.85) projected
  line L22 (-18, -1.85) -> (-2.5, -1.85) projected
  line L23 (-2.5, -1.85) -> (-2.5, -46.05) projected
  line L24 (-14.3503, 16.6891) -> (-3.9031, 19.0008) projected
  line L25 (-3.9031, 19.0008) -> (-3.5574, 17.4386) projected
  line L26 (-3.5574, 17.4386) -> (-14.0047, 15.1269) projected
  line L27 (-14.0047, 15.1269) -> (-14.3503, 16.6891) projected
  line L28 (-1.2105, 19.0122) -> (9.235, 16.6922) projected
  line L29 (9.235, 16.6922) -> (8.888, 15.1302) projected
  line L30 (8.888, 15.1302) -> (-1.5574, 17.4503) projected
  line L31 (-1.5574, 17.4503) -> (-1.2105, 19.0122) projected
  line L32 (31.4357, 13.9645) -> (32.5559, 15.107) projected
  line L33 (32.5559, 15.107) -> (40.1958, 7.6154) projected
  line L34 (40.1958, 7.6154) -> (39.0755, 6.473) projected
  line L35 (39.0755, 6.473) -> (31.4357, 13.9645) projected
  line L36 (-38.6369, 1.9142) -> (-39.7739, 3.0399) projected
  line L37 (-39.7739, 3.0399) -> (-32.2458, 10.6437) projected
  line L38 (-32.2458, 10.6437) -> (-31.1088, 9.5181) projected
  line L39 (-31.1088, 9.5181) -> (-38.6369, 1.9142) projected
  line L40 (34.6166, 1.9821) -> (36.1788, 2.3275) projected
  line L41 (36.1788, 2.3275) -> (38.4885, -8.1203) projected
  line L42 (38.4885, -8.1203) -> (36.9263, -8.4656) projected
  line L43 (36.9263, -8.4656) -> (34.6166, 1.9821) projected
  line L44 (-39.2388, -12.6185) -> (-40.8006, -12.2713) projected
  line L45 (-40.8006, -12.2713) -> (-38.4785, -1.8263) projected
  line L46 (-38.4785, -1.8263) -> (-36.9167, -2.1735) projected
  line L47 (-36.9167, -2.1735) -> (-39.2388, -12.6185) projected
  circle A2 centre (-38.1278, 33.4973) radius 3 projected
  circle A3 centre (38.1278, 33.4973) radius 3 projected
  circle A4 centre (21.5, -6.85) radius 1.5 projected
  circle A5 centre (-21.5, -6.85) radius 1.5 projected
  circle A6 centre (-7.5, -24.85) radius 1.75 projected
  circle A7 centre (7.5, -24.85) radius 1.75 projected
  line L48 (50, 39.3049) -> (-50, 39.3049) projected
  line L49 (-50, 39.3049) -> (-50, -15.75) projected
  line L50 (-50, -15.75) -> (-15, -15.75) projected
  line L51 (-15, -15.75) -> (-15, -33.85) projected
  line L52 (-15, -33.85) -> (15, -33.85) projected
  line L53 (15, -33.85) -> (15, -15.75) projected
  line L54 (15, -15.75) -> (50, -15.75) projected
  line L55 (50, -15.75) -> (50, 39.3049) projected
  circle A8 centre (7.5, -6.85) radius 1.5 projected
  circle A9 centre (-7.5, -6.85) radius 1.5 projected
  line L56 (-18, -1.85) -> (-41, -1.85)
  line L57 (-41, -1.85) -> (-41, -15.75)
  line L58 (-41, -15.75) -> (-18, -15.75)
  line L59 (-18, -15.75) -> (-18, -1.85)
  line L60 (-41, -1.85) -> (-18, -1.85)
  line L61 (-18, -1.85) -> (-18, -14.85)
  line L62 (-18, -14.85) -> (-41, -14.85)
  line L63 (-41, -14.85) -> (-41, -1.85)
  line L64 (41, -13.0168) -> (41, 17.8601) projected
  line L65 (41, -1.85) -> (18.1665, -1.85)
  line L66 (18.1665, -1.85) -> (18.1665, -14.85)
  line L67 (18.1665, -14.85) -> (41, -14.85)
  line L68 (41, -14.85) -> (41, -1.85)
  line L69 (18, -13.0168) -> (18.1665, -13.0168)
  line L70 (18.1665, -13.0168) -> (18.1665, -14.85)
  line L71 (18.1665, -14.85) -> (18, -14.85)
  line L72 (18, -14.85) -> (18, -13.0168)
  point P0 (0, 0)
  point P1 (-18, -13.0168)
  point P2 (-41, -13.0168)
  dimension "d51" = 13
  constraints: 32 end point, 8 parallel, 6 point on line, 4 horizontal, 4 perpendicular
  measures "d51" distance of L60.end L61.end
extrude "Extrusion17" add sketch "Sketch17" against normal blind 2 contours L59 L62 L57 L20 | L4 L66 L71 L72 | L4 L68 L67 L66
sketch "Sketch18" plane through (0, 0, 2.4) normal (0, 0, 1) x (1, 0, 0)
  circle A0 centre (-21.5, -6.85) radius 1.5 projected
  circle A1 centre (21.5, -6.85) radius 1.5 projected
  line L0 (-2.5, -46.05) -> (2.5, -46.05) projected
  line L1 (2.5, -46.05) -> (2.5, -1.85) projected
  line L2 (2.5, -1.85) -> (18, -1.85) projected
  line L3 (18, -1.85) -> (18, -14.85) projected
  line L4 (18, -14.85) -> (41, -14.85) projected
  line L5 (41, -14.85) -> (41, 17.8601) projected
  line L6 (41, 17.8601) -> (35.2556, 17.8601) projected
  line L7 (35.2556, 17.8601) -> (35.2556, 28.0794) projected
  line L8 (35.2556, 28.0794) -> (41, 28.0794) projected
  line L9 (41, 28.0794) -> (41, 36.1074) projected
  line L10 (41, 36.1074) -> (28, 36.1074) projected
  line L11 (28, 36.1074) -> (28, 28.0794) projected
  line L12 (28, 28.0794) -> (-28, 28.0794) projected
  line L13 (-28, 28.0794) -> (-28, 36.1074) projected
  line L14 (-28, 36.1074) -> (-41, 36.1074) projected
  line L15 (-41, 36.1074) -> (-41, 28.0794) projected
  line L16 (-41, 28.0794) -> (-35.2556, 28.0794) projected
  line L17 (-35.2556, 28.0794) -> (-35.2556, 17.8601) projected
  line L18 (-35.2556, 17.8601) -> (-41, 17.8601) projected
  line L19 (-41, 17.8601) -> (-41, -14.85) projected
  line L20 (-41, -14.85) -> (-18, -14.85) projected
  line L21 (-18, -14.85) -> (-18, -1.85) projected
  line L22 (-18, -1.85) -> (-2.5, -1.85) projected
  line L23 (-2.5, -1.85) -> (-2.5, -46.05) projected
  line L24 (-14.3503, 16.6891) -> (-3.9031, 19.0008) projected
  line L25 (-3.9031, 19.0008) -> (-3.5574, 17.4386) projected
  line L26 (-3.5574, 17.4386) -> (-14.0047, 15.1269) projected
  line L27 (-14.0047, 15.1269) -> (-14.3503, 16.6891) projected
  line L28 (-1.2105, 19.0122) -> (9.235, 16.6922) projected
  line L29 (9.235, 16.6922) -> (8.888, 15.1302) projected
  line L30 (8.888, 15.1302) -> (-1.5574, 17.4503) projected
  line L31 (-1.5574, 17.4503) -> (-1.2105, 19.0122) projected
  line L32 (31.4357, 13.9645) -> (32.5559, 15.107) projected
  line L33 (32.5559, 15.107) -> (40.1958, 7.6154) projected
  line L34 (40.1958, 7.6154) -> (39.0755, 6.473) projected
  line L35 (39.0755, 6.473) -> (31.4357, 13.9645) projected
  line L36 (-38.6369, 1.9142) -> (-39.7739, 3.0399) projected
  line L37 (-39.7739, 3.0399) -> (-32.2458, 10.6437) projected
  line L38 (-32.2458, 10.6437) -> (-31.1088, 9.5181) projected
  line L39 (-31.1088, 9.5181) -> (-38.6369, 1.9142) projected
  line L40 (34.6166, 1.9821) -> (36.1788, 2.3275) projected
  line L41 (36.1788, 2.3275) -> (38.4885, -8.1203) projected
  line L42 (38.4885, -8.1203) -> (36.9263, -8.4656) projected
  line L43 (36.9263, -8.4656) -> (34.6166, 1.9821) projected
  line L44 (-39.2388, -12.6185) -> (-40.8006, -12.2713) projected
  line L45 (-40.8006, -12.2713) -> (-38.4785, -1.8263) projected
  line L46 (-38.4785, -1.8263) -> (-36.9167, -2.1735) projected
  line L47 (-36.9167, -2.1735) -> (-39.2388, -12.6185) projected
  line L48 (-28, 36.1074) -> (-28, 28.0794) projected
  line L49 (-41, 28.0794) -> (-41, 36.1074) projected
  line L50 (-28, 28.0794) -> (-41, 28.0794)
  line L51 (-41, 28.0794) -> (-41, 36.0794)
  line L52 (-41, 36.0794) -> (-28, 36.0794)
  line L53 (-28, 36.0794) -> (-28, 28.0794)
  line L54 (-41, 28.0794) -> (-35, 28.0794)
  line L55 (-35, 28.0794) -> (-35, 17.0794)
  line L56 (-35, 17.0794) -> (-41, 17.0794)
  line L57 (-41, 17.0794) -> (-41, 28.0794)
  line L58 (28, 36.1074) -> (28, 28.0794) projected
  line L59 (-28, -1.8263) -> (28, -1.8263)
  line L60 (28, -1.8263) -> (28, 28.1737)
  line L61 (28, 28.1737) -> (-28, 28.1737)
  line L62 (-28, 28.1737) -> (-28, -1.8263)
  line L63 (0, 0) -> (0, 28.1737)
  line L64 (28, 36.1074) -> (41, 36.1074)
  line L65 (41, 28.0794) -> (35.2556, 28.0794)
  line L66 (35.2556, 28.0794) -> (35.2556, 17.8601)
  line L67 (28, 28.0794) -> (41, 28.0794)
  line L68 (41, 28.0794) -> (41, 36.0794)
  line L69 (28, 36.0794) -> (28, 28.0794)
  line L70 (35, 17.0794) -> (41, 17.0794)
  line L71 (41, 17.0794) -> (41, 28.0794)
  line L72 (28, -1.8263) -> (-28, -1.8263)
  line L73 (-28, 28.1737) -> (28, 28.1737)
  line L74 (28, 28.1737) -> (28, -1.8263)
  point P0 (41, 17.8601)
  point P1 (0, 28.0794)
  dimension "d54" = 8
  dimension "d55" = 6
  dimension "d56" = 11
  dimension "d57" = 30
  constraints: 48 end point, 10 symmetric about line, 6 parallel, 3 horizontal, 3 perpendicular, 2 point on line, 1 midpoint
  measures "d54" distance of L50.end L51.end
  measures "d55" distance of L55.end L56.end
  measures "d56" distance of L54.end L55.end
  measures "d57" distance of L60.end L59.end
extrude "Extrusion18" cut sketch "Sketch18" against normal blind 2 contours L19 L18 L17 L50 L55 L56 | L57 L16 L17 L18 | L6 L7 L8 L71
extrude "Extrusion19" add sketch "Sketch18" against normal blind 2 contours L13 L61 L63 L12
sketch "Sketch19" plane through (0, 0, 2.4) normal (0, 0, 1) x (1, 0, 0)
  line L0 (-39.2388, -12.6185) -> (-40.8006, -12.2713) projected
  line L1 (-40.8006, -12.2713) -> (-38.4785, -1.8263) projected
  line L2 (-38.4785, -1.8263) -> (-36.9167, -2.1735) projected
  line L3 (-36.9167, -2.1735) -> (-39.2388, -12.6185) projected
  line L4 (34.6166, 1.9821) -> (36.1788, 2.3275) projected
  line L5 (36.1788, 2.3275) -> (38.4885, -8.1203) projected
  line L6 (38.4885, -8.1203) -> (36.9263, -8.4656) projected
  line L7 (36.9263, -8.4656) -> (34.6166, 1.9821) projected
  line L8 (-38.6369, 1.9142) -> (-39.7739, 3.0399) projected
  line L9 (-39.7739, 3.0399) -> (-32.2458, 10.6437) projected
  line L10 (-32.2458, 10.6437) -> (-31.1088, 9.5181) projected
  line L11 (-31.1088, 9.5181) -> (-38.6369, 1.9142) projected
  line L12 (31.4357, 13.9645) -> (32.5559, 15.107) projected
  line L13 (32.5559, 15.107) -> (40.1958, 7.6154) projected
  line L14 (40.1958, 7.6154) -> (39.0755, 6.473) projected
  line L15 (39.0755, 6.473) -> (31.4357, 13.9645) projected
  line L16 (-1.2105, 19.0122) -> (9.235, 16.6922) projected
  line L17 (9.235, 16.6922) -> (8.888, 15.1302) projected
  line L18 (8.888, 15.1302) -> (-1.5574, 17.4503) projected
  line L19 (-1.5574, 17.4503) -> (-1.2105, 19.0122) projected
  line L20 (-14.3503, 16.6891) -> (-3.9031, 19.0008) projected
  line L21 (-3.9031, 19.0008) -> (-3.5574, 17.4386) projected
  line L22 (-3.5574, 17.4386) -> (-14.0047, 15.1269) projected
  line L23 (-14.0047, 15.1269) -> (-14.3503, 16.6891) projected
  line L24 (-41, 28.0794) -> (-35, 28.0794) projected
  line L25 (-35, 28.0794) -> (-35, 17.0794) projected
  line L26 (-35, 17.0794) -> (-41, 17.0794) projected
  line L27 (-41, 17.0794) -> (-41, -14.85) projected
  line L28 (-41, -14.85) -> (-18, -14.85) projected
  line L29 (-18, -14.85) -> (-18, -1.85) projected
  line L30 (-18, -1.85) -> (-2.5, -1.85) projected
  line L31 (-2.5, -1.85) -> (-2.5, -46.05) projected
  line L32 (-2.5, -46.05) -> (2.5, -46.05) projected
  line L33 (2.5, -46.05) -> (2.5, -1.85) projected
  line L34 (2.5, -1.85) -> (18, -1.85) projected
  line L35 (18, -1.85) -> (18, -14.85) projected
  line L36 (18, -14.85) -> (41, -14.85) projected
  line L37 (41, -14.85) -> (41, 17.8601) projected
  line L38 (41, 17.8601) -> (35.2556, 17.8601) projected
  line L39 (35.2556, 17.8601) -> (35.2556, 28.0794) projected
  line L40 (35.2556, 28.0794) -> (41, 28.0794) projected
  line L41 (41, 28.0794) -> (41, 36.1074) projected
  line L42 (41, 36.1074) -> (28, 36.1074) projected
  line L43 (28, 36.1074) -> (28, 28.0794) projected
  line L44 (28, 28.0794) -> (0, 28.0794) projected
  line L45 (0, 28.0794) -> (0, 28.1737) projected
  line L46 (0, 28.1737) -> (-28, 28.1737) projected
  line L47 (-28, 28.1737) -> (-28, 36.1074) projected
  line L48 (-28, 36.1074) -> (-41, 36.1074) projected
  line L49 (-41, 36.1074) -> (-41, 28.0794) projected
  circle A0 centre (21.5, -6.85) radius 1.5 projected
  circle A1 centre (-21.5, -6.85) radius 1.5 projected
  line L50 (-41, 17.0794) -> (41, 17.0794)
  line L51 (41, 17.8601) -> (41, -14.85) projected
  line L52 (35.2556, 17.8601) -> (41, 17.8601) projected
  line L53 (35.2556, 17.8601) -> (35.2556, 10.2188)
  point P0 (0, 0)
  point P1 (35.2556, 17.0794)
  constraints: 4 end point, 2 point on line, 1 midpoint, 1 perpendicular
extrude "Extrusion20" cut sketch "Sketch19" against normal blind 2 contours L53 L38 L37 L50
sketch "Sketch20" plane through (0, 0, 2.4) normal (0, 0, 1) x (1, 0, 0)
  line L0 (0, 0) -> (0, 62.7623)
  line L1 (35.2556, 17.0794) -> (35.2556, 28.0794) projected
  line L2 (35.2556, 28.0794) -> (41, 28.0794) projected
  line L3 (41, 28.0794) -> (41, 36.1074) projected
  line L4 (41, 36.1074) -> (28, 36.1074) projected
  line L5 (28, 36.1074) -> (28, 28.0794) projected
  line L6 (28, 28.0794) -> (0, 28.0794) projected
  line L7 (0, 28.0794) -> (0, 28.1737) projected
  line L8 (0, 28.1737) -> (-28, 28.1737) projected
  line L9 (-28, 28.1737) -> (-28, 36.1074) projected
  line L10 (-28, 36.1074) -> (-41, 36.1074) projected
  line L11 (-41, 36.1074) -> (-41, 28.0794) projected
  line L12 (-41, 28.0794) -> (-35, 28.0794) projected
  line L13 (-35, 28.0794) -> (-35, 17.0794) projected
  line L14 (-35, 17.0794) -> (-41, 17.0794) projected
  line L15 (-41, 17.0794) -> (-41, -14.85) projected
  line L16 (-41, -14.85) -> (-18, -14.85) projected
  line L17 (-18, -14.85) -> (-18, -1.85) projected
  line L18 (-18, -1.85) -> (-2.5, -1.85) projected
  line L19 (-2.5, -1.85) -> (-2.5, -46.05) projected
  line L20 (-2.5, -46.05) -> (2.5, -46.05) projected
  line L21 (2.5, -46.05) -> (2.5, -1.85) projected
  line L22 (2.5, -1.85) -> (18, -1.85) projected
  line L23 (18, -1.85) -> (18, -14.85) projected
  line L24 (18, -14.85) -> (41, -14.85) projected
  line L25 (41, -14.85) -> (41, 17.0794) projected
  line L26 (41, 17.0794) -> (35.2556, 17.0794) projected
  line L27 (-39.2388, -12.6185) -> (-40.8006, -12.2713) projected
  line L28 (-40.8006, -12.2713) -> (-38.4785, -1.8263) projected
  line L29 (-38.4785, -1.8263) -> (-36.9167, -2.1735) projected
  line L30 (-36.9167, -2.1735) -> (-39.2388, -12.6185) projected
  line L31 (34.6166, 1.9821) -> (36.1788, 2.3275) projected
  line L32 (36.1788, 2.3275) -> (38.4885, -8.1203) projected
  line L33 (38.4885, -8.1203) -> (36.9263, -8.4656) projected
  line L34 (36.9263, -8.4656) -> (34.6166, 1.9821) projected
  line L35 (-38.6369, 1.9142) -> (-39.7739, 3.0399) projected
  line L36 (-39.7739, 3.0399) -> (-32.2458, 10.6437) projected
  line L37 (-32.2458, 10.6437) -> (-31.1088, 9.5181) projected
  line L38 (-31.1088, 9.5181) -> (-38.6369, 1.9142) projected
  line L39 (31.4357, 13.9645) -> (32.5559, 15.107) projected
  line L40 (32.5559, 15.107) -> (40.1958, 7.6154) projected
  line L41 (40.1958, 7.6154) -> (39.0755, 6.473) projected
  line L42 (39.0755, 6.473) -> (31.4357, 13.9645) projected
  line L43 (-1.2105, 19.0122) -> (9.235, 16.6922) projected
  line L44 (9.235, 16.6922) -> (8.888, 15.1302) projected
  line L45 (8.888, 15.1302) -> (-1.5574, 17.4503) projected
  line L46 (-1.5574, 17.4503) -> (-1.2105, 19.0122) projected
  line L47 (-14.3503, 16.6891) -> (-3.9031, 19.0008) projected
  line L48 (-3.9031, 19.0008) -> (-3.5574, 17.4386) projected
  line L49 (-3.5574, 17.4386) -> (-14.0047, 15.1269) projected
  line L50 (-14.0047, 15.1269) -> (-14.3503, 16.6891) projected
  circle A0 centre (21.5, -6.85) radius 1.5 projected
  circle A1 centre (-21.5, -6.85) radius 1.5 projected
  line L51 (-1.2105, 19.0122) -> (-35, 19.0122)
  line L52 (-35, 28.0794) -> (-35, 17.0794) projected
  line L53 (-35, 19.0122) -> (35.2556, 19.0122)
  constraints: 6 end point, 3 point on line, 1 perpendicular, 1 vertical
sketch "Sketch21" plane through (0, 0, 2.4) normal (0, 0, 1) x (1, 0, 0)
  line L0 (35.2556, 17.0794) -> (35.2556, 28.0794) projected
  line L1 (35.2556, 28.0794) -> (41, 28.0794) projected
  line L2 (41, 28.0794) -> (41, 36.1074) projected
  line L3 (41, 36.1074) -> (28, 36.1074) projected
  line L4 (28, 36.1074) -> (28, 28.0794) projected
  line L5 (28, 28.0794) -> (0, 28.0794) projected
  line L6 (0, 28.0794) -> (0, 28.1737) projected
  line L7 (0, 28.1737) -> (-28, 28.1737) projected
  line L8 (-28, 28.1737) -> (-28, 36.1074) projected
  line L9 (-28, 36.1074) -> (-41, 36.1074) projected
  line L10 (-41, 36.1074) -> (-41, 28.0794) projected
  line L11 (-41, 28.0794) -> (-35, 28.0794) projected
  line L12 (-35, 28.0794) -> (-35, 17.0794) projected
  line L13 (-35, 17.0794) -> (-41, 17.0794) projected
  line L14 (-41, 17.0794) -> (-41, -14.85) projected
  line L15 (-41, -14.85) -> (-18, -14.85) projected
  line L16 (-18, -14.85) -> (-18, -1.85) projected
  line L17 (-18, -1.85) -> (-2.5, -1.85) projected
  line L18 (-2.5, -1.85) -> (-2.5, -46.05) projected
  line L19 (-2.5, -46.05) -> (2.5, -46.05) projected
  line L20 (2.5, -46.05) -> (2.5, -1.85) projected
  line L21 (2.5, -1.85) -> (18, -1.85) projected
  line L22 (18, -1.85) -> (18, -14.85) projected
  line L23 (18, -14.85) -> (41, -14.85) projected
  line L24 (41, -14.85) -> (41, 17.0794) projected
  line L25 (41, 17.0794) -> (35.2556, 17.0794) projected
  line L26 (-39.2388, -12.6185) -> (-40.8006, -12.2713) projected
  line L27 (-40.8006, -12.2713) -> (-38.4785, -1.8263) projected
  line L28 (-38.4785, -1.8263) -> (-36.9167, -2.1735) projected
  line L29 (-36.9167, -2.1735) -> (-39.2388, -12.6185) projected
  line L30 (34.6166, 1.9821) -> (36.1788, 2.3275) projected
  line L31 (36.1788, 2.3275) -> (38.4885, -8.1203) projected
  line L32 (38.4885, -8.1203) -> (36.9263, -8.4656) projected
  line L33 (36.9263, -8.4656) -> (34.6166, 1.9821) projected
  line L34 (-38.6369, 1.9142) -> (-39.7739, 3.0399) projected
  line L35 (-39.7739, 3.0399) -> (-32.2458, 10.6437) projected
  line L36 (-32.2458, 10.6437) -> (-31.1088, 9.5181) projected
  line L37 (-31.1088, 9.5181) -> (-38.6369, 1.9142) projected
  line L38 (31.4357, 13.9645) -> (32.5559, 15.107) projected
  line L39 (32.5559, 15.107) -> (40.1958, 7.6154) projected
  line L40 (40.1958, 7.6154) -> (39.0755, 6.473) projected
  line L41 (39.0755, 6.473) -> (31.4357, 13.9645) projected
  line L42 (-1.2105, 19.0122) -> (9.235, 16.6922) projected
  line L43 (9.235, 16.6922) -> (8.888, 15.1302) projected
  line L44 (8.888, 15.1302) -> (-1.5574, 17.4503) projected
  line L45 (-1.5574, 17.4503) -> (-1.2105, 19.0122) projected
  line L46 (-14.3503, 16.6891) -> (-3.9031, 19.0008) projected
  line L47 (-3.9031, 19.0008) -> (-3.5574, 17.4386) projected
  line L48 (-3.5574, 17.4386) -> (-14.0047, 15.1269) projected
  line L49 (-14.0047, 15.1269) -> (-14.3503, 16.6891) projected
  circle A0 centre (21.5, -6.85) radius 1.5 projected
  circle A1 centre (-21.5, -6.85) radius 1.5 projected
  line L50 (28, 36.1074) -> (28, 28.0794) projected
  line L51 (-28, 28.1737) -> (-28, 36.1074) projected
  line L52 (28, 36.1074) -> (-28, 36.1074)
  line L53 (-28, 36.1074) -> (-28, 28.1737)
  line L54 (-28, 28.1737) -> (28, 28.1737)
  line L55 (28, 28.1737) -> (28, 36.1074)
  point P0 (0, 0)
  constraints: 8 end point, 2 parallel, 1 horizontal, 1 perpendicular
extrude "Extrusion21" add sketch "Sketch21" against normal blind 2 contours L4 L5 L6 L54
sketch "Sketch22" plane through (0, 0, 2.4) normal (0, 0, 1) x (1, 0, 0)
  line L0 (-28, 28.1737) -> (28, 28.1737) projected
  line L1 (0, 28.1737) -> (7, 28.1737)
  line L2 (7, 28.1737) -> (7, 22.8553)
  line L3 (7, 22.8553) -> (0, 22.8553)
  line L4 (0, 22.8553) -> (0, 28.1737)
  line L5 (7, 22.8553) -> (-7, 22.8553)
  line L6 (-7, 22.8553) -> (-7, 28.1737)
  line L7 (-7, 28.1737) -> (7, 28.1737)
  line L8 (7, 28.1737) -> (7, 22.8553)
  point P0 (0, 0)
  dimension "d66" = 7
  dimension "d67" = 14
  constraints: 16 end point, 4 parallel, 2 horizontal, 2 perpendicular, 1 midpoint, 1 point on line
  measures "d66" distance of L2.end L3.end
  measures "d67" distance of L6.end L7.end
extrude "Extrusion22" add sketch "Sketch22" along normal blind 10
extrude "Extrusion23" add sketch "Sketch20" against normal blind 2 contours L43 L44 L45 L0 | L0 L45 L46 L43 | L27 L28 L29 L30 | L31 L32 L33 L34 | L35 L36 L37 L38 | L39 L40 L41 L42 | L47 L48 L49 L50
sketch "Sketch23" plane through (0, 0, 2.4) normal (0, 0, 1) x (1, 0, 0)
  point P0 (0, 0)